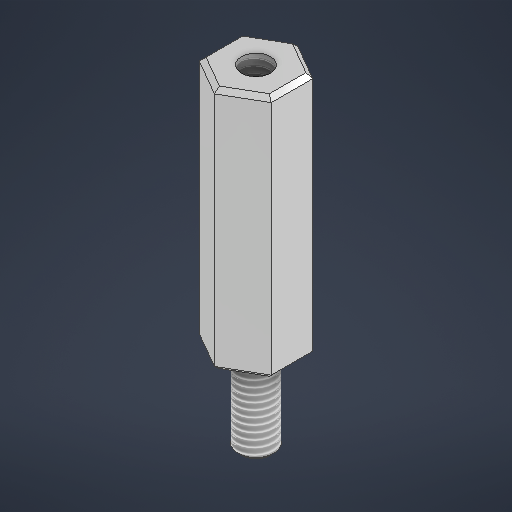
# Autodesk Inventor part: Abstandsbolzen 17mm
Saved by Autodesk Inventor 2025.2 (Build 292293000, 293)
## iProperties
Created: 2024-05-14
Part Number: Abstandsbolzen 17mm
Material: Generisch
Document SubType Name: Modeling
Designer: Fabian
Density: 1 g/cm^3
Appearance: Aluminium - poliert
Author: Fabian
Autodesk Inventor part; units mm, degrees
ref_plane "YZ Plane" through (0, 0, 0) normal (1, 0, 0) x (0, 1, 0)
ref_plane "XZ Plane" through (0, 0, 0) normal (0, 1, 0) x (-1, 0, 0)
ref_plane "XY Plane" through (0, 0, 0) normal (0, 0, 1) x (1, 0, 0)
sketch "Skizze1" plane through (0, 0, 0) normal (0, 1, 0) x (-1, 0, 0)
  line L0 (2.5, -1.4434) -> (0, -2.8868)
  line L1 (0, -2.8868) -> (-2.5, -1.4434)
  line L2 (-2.5, -1.4434) -> (-2.5, 1.4434)
  line L3 (-2.5, 1.4434) -> (0, 2.8868)
  line L4 (0, 2.8868) -> (2.5, 1.4434)
  line L5 (2.5, 1.4434) -> (2.5, -1.4434)
  point P0 (0, 0)
  point P1 (0, 0)
  point P2 (0, 0)
  dimension "d0" = 5
  constraints: 12 end point, 2 coincident, 13 other
  measures "d0" distance between parallel lines of L2 L5
extrude "Extrusion1" add sketch "Skizze1" against normal blind 17
hole "Bohrung1" at (0, 0, 0) direction (0, -1, 0) diameter 2.013 depth 8 tip angle 118 thread size "M2.5x0.45" class "6H" standard "ISO Metric profile"
sketch "Skizze2" plane through (0, -17, 0) normal (0, -1, 0) x (1, 0, 0)
  circle A0 centre (0, 0) radius 1.0065 projected
  circle A1 centre (0, 0) radius 1.25
  dimension "d10" = 2.5
  constraints: 1 centre point, 1 coincident
  measures "d10" diameter of A1
extrude "Extrusion2" add sketch "Skizze2" along normal blind 6 contours A0 | A1
thread "Gewinde1" size "M2.5x0.45" class "6g" standard "ISO Metric profile" full length
chamfer "Fasen1" distance 0.25 angle 45 1 edges at (-1.25, -23, 0)
chamfer "Fasen2" distance 0.3 angle 45 12 edges at (2.5, 0, 0) (1.25, 0, 2.1651) (-1.25, 0, 2.1651) (-2.5, 0, 0) (-1.25, 0, -2.1651) (1.25, 0, -2.1651) (2.5, -17, 0) (1.25, -17, 2.1651) (-1.25, -17, 2.1651) (-2.5, -17, 0) (-1.25, -17, -2.1651) (1.25, -17, -2.1651)
